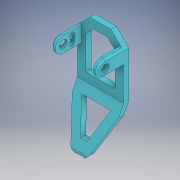
# Autodesk Inventor part: TIBIA
Saved by Autodesk Inventor 2017 (Build 210142000, 142)
## iProperties
Created: 2017-09-24
Part Number: TIBIA
Material: Generic
Document SubType Name: Modeling
Designer: Alexander Miller
Density: 1 g/cm^3
Appearance: Cadet Blue
Author: Alexander Miller
Autodesk Inventor part; units mm, degrees
ref_plane "YZ Plane" through (0, 0, 0) normal (1, 0, 0) x (0, 1, 0)
ref_plane "XZ Plane" through (0, 0, 0) normal (0, 1, 0) x (-1, 0, 0)
ref_plane "XY Plane" through (0, 0, 0) normal (0, 0, 1) x (1, 0, 0)
sketch "Sketch7" plane through (0, 0, 0) normal (0, 1, 0) x (-1, 0, 0)
  line L0 (-15, 22) -> (15, 22)
  line L1 (15, 22) -> (15, -22)
  line L2 (15, -22) -> (-15, -22)
  line L3 (-15, -22) -> (-15, 22)
  line L4 (-10, 18) -> (15, 18)
  line L5 (15, 18) -> (15, -18)
  line L6 (15, -18) -> (-10, -18)
  line L7 (-10, -18) -> (-10, 18)
  point P0 (0, 0)
  point P1 (0, -22)
  point P2 (15, 0)
  point P3 (15, 0)
  dimension "d32" = 4
  dimension "d33" = 5
  dimension "d35" = 44
  dimension "d36" = 25
  constraints: 16 end point, 4 parallel, 3 midpoint, 2 horizontal, 2 horizontal alignment, 2 perpendicular, 1 collinear, 1 vertical alignment
  measures "d32" distance between parallel lines of L0 L4
  measures "d33" distance between parallel lines of L3 L7
  measures "d35" distance of L0.end L1.end
  measures "d36" distance between parallel lines of L7 L1
extrude "Extrusion7" add sketch "Sketch7" along normal blind 15 contours L0 L1 L4 L7 L6 L2 L3
fillet "Fillet4" radius 7.5 4 edges at (-15, 15, 20) (-15, 15, -20) (-15, 0, 20) (-15, 0, -20)
sketch "Sketch8" plane through (15, 0, 22) normal (0, 0, 1) x (1, 0, 0)
  circle A0 centre (-22.5, 7.5) radius 3.675
  arc A1 (-22.5, 15) -> (-22.5, 0) centre (-22.5, 7.5) ccw projected
  point P0 (-15, 0)
  dimension "d40" = 7.35
  constraints: 1 centre point, 1 concentric
  measures "d40" diameter of A0
extrude "Extrusion8" cut sketch "Sketch8" against normal up to surface (4 mm away)
sketch "Sketch9" plane through (15, 0, -22) normal (0, 0, -1) x (-1, 0, 0)
  circle A0 centre (22.5, 7.5) radius 3.75
  arc A1 (22.5, 0) -> (22.5, 15) centre (22.5, 7.5) ccw projected
  point P0 (15, 0)
  dimension "d43" = 7.5
  constraints: 1 centre point, 1 concentric
  measures "d43" diameter of A0
extrude "Extrusion9" cut sketch "Sketch9" against normal up to surface (4 mm away)
sketch "Sketch10" plane through (15, 0, -22) normal (0, 0, -1) x (-1, 0, 0)
  line L0 (22.5, 3.75) -> (5.5, 3.75)
  line L1 (5.5, 3.75) -> (5.5, 11.25)
  line L2 (5.5, 11.25) -> (22.5, 11.25)
  circle A0 centre (22.5, 7.5) radius 3.75 projected
  point P0 (15, 0)
  dimension "d47" = 17
  constraints: 6 end point, 2 perpendicular, 2 point on circle, 2 tangent, 1 horizontal
  measures "d47" distance from line of A0.centre L1
extrude "Extrusion10" cut sketch "Sketch10" against normal blind 2 contours L0 L1 L2 A0
fillet "Fillet5" radius 1.75 2 edges at (9.5, 11.25, -21) (9.5, 3.75, -21)
sketch "Sketch12" plane through (15, 0, 22) normal (0, 0, 1) x (1, 0, 0)
  line L0 (-5, 0) -> (-5, 15) projected
  line L1 (0, 0) -> (0, 15) projected
  line L2 (-5, 25) -> (0, 25)
  line L3 (0, 25) -> (0, -30)
  line L4 (0, -30) -> (-5, -30)
  line L5 (-5, -30) -> (-5, 25)
  line L6 (-22.5, 15) -> (0, 15) projected
  line L7 (0, 0) -> (-22.5, 0) projected
  line L8 (-5, -30) -> (-25, -70.9989)
  line L9 (-25, -70.9989) -> (-20, -70.9989)
  line L10 (-20, -70.9989) -> (0, -30)
  arc A0 (-25, -70.9989) -> (-20, -70.9989) centre (-22.5, -72.2184) ccw
  point P0 (-15, 0)
  point P1 (-22.5, -70.9989)
  dimension "d57" = 10
  dimension "d60" = 100
  dimension "d62" = 30
  constraints: 14 end point, 3 parallel, 2 collinear, 2 horizontal, 2 point on circle, 1 centre point, 1 midpoint, 1 perpendicular, 1 tangent
  measures "d57" distance between parallel lines of L6 L2
  measures "d62" distance between parallel lines of L7 L4
extrude "Extrusion11" add sketch "Sketch12" against normal up to surface (44 mm away) contours L7 L3 L4 L5 | L5 L2 L3 L6 | L4 L10 L9 L8 | L9 A0
chamfer "Chamfer8" distance 12 angle 45 2 edges at (12.5, 25, 22) (12.5, 25, -22)
chamfer "Chamfer9" distance 2 angle 45 4 edges at (-14.3736, 10.5007, 22) (1.25, 0, 22) (-14.3736, 10.5007, -22) (1.25, 0, -22)
sketch "Sketch15" plane through (15, -30, 22) normal (1, 0, 0) x (0, 0, -1)
  line L0 (-4.3749, 0) -> (48.3749, 0)
  line L1 (48.3749, 0) -> (48.3749, -54.3582)
  line L2 (48.3749, -54.3582) -> (-4.3749, -54.3582)
  line L3 (-4.3749, -54.3582) -> (-4.3749, 0)
  line L4 (0, 0) -> (44, 0) projected
  circle A0 centre (22, -35) radius 10
  line L5 (-4.3749, 0) -> (12.8511, -39.0371)
  line L6 (48.3749, 0) -> (31.1489, -39.0371)
  line L7 (12, 55) -> (32, 55) projected
  line L8 (0, -45) -> (44, -45) projected
  point P0 (22, 55)
  point P1 (22, 0)
  point P2 (22, 55)
  dimension "d78" = 20
  constraints: 12 end point, 3 midpoint, 3 tangent, 2 parallel, 2 point on circle, 2 vertical alignment, 1 centre point, 1 collinear, 1 horizontal, 1 perpendicular
  measures "d78" diameter of A0
extrude "Extrusion13" cut sketch "Sketch15" against normal through all contours L5 A0 L6 L1 L2 L3
sketch "Sketch16" plane through (15, -30, 22) normal (1, 0, 0) x (0, 0, -1)
  line L0 (32, 55) -> (44, 43) projected
  line L1 (12, 55) -> (32, 55) projected
  line L2 (0, 43) -> (12, 55) projected
  line L3 (0, 0) -> (0, 43) projected
  line L4 (0, 0) -> (44, 0) projected
  line L5 (44, 0) -> (44, 43) projected
  line L6 (31.1489, -39.0371) -> (44, -9.9143) projected
  line L7 (44, -9.9143) -> (44, 0) projected
  line L8 (0, 0) -> (44, 0) projected
  line L9 (0, -9.9143) -> (0, 0) projected
  line L10 (0, -9.9143) -> (12.8511, -39.0371) projected
  arc A0 (12.8511, -39.0371) -> (13.9991, -40.9989) centre (22, -35) ccw projected
  line L11 (13.9991, -40.9989) -> (30.0009, -40.9989) projected
  arc A1 (30.0009, -40.9989) -> (31.1489, -39.0371) centre (22, -35) ccw projected
  line L12 (15.3137, 47) -> (28.6863, 47)
  line L13 (28.6863, 47) -> (36, 39.6863)
  line L14 (36, 39.6863) -> (36, 8)
  line L15 (36, 8) -> (8, 8)
  line L16 (8, 8) -> (8, 39.6863)
  line L17 (8, 39.6863) -> (15.3137, 47)
  line L18 (18.9309, -32.9989) -> (8, -8.2276)
  line L19 (8, -8.2276) -> (8, -8)
  line L20 (8, -8) -> (36, -8)
  line L21 (36, -8) -> (36, -8.2276)
  line L22 (36, -8.2276) -> (25.0691, -32.9989)
  line L23 (25.0691, -32.9989) -> (18.9309, -32.9989)
  line L24 (8, 8) -> (36, 8)
  line L25 (36, 8) -> (36, -8)
  line L26 (36, -8) -> (8, -8)
  line L27 (8, -8) -> (8, 8)
  point P0 (22, 30)
  dimension "d81" = 8
  constraints: 32 end point, 4 collinear, 2 parallel, 1 horizontal, 1 perpendicular, 1 vertical alignment, 10 other
  measures "d81" distance between parallel lines of L3 L16
extrude "Extrusion14" cut sketch "Sketch16" against normal through all contours L15 L16 L17 L12 L13 L14 | L21 L22 L23 L18 L19 L20
sketch "Sketch17" plane through (10, 0, 18) normal (0, 0, -1) x (-1, 0, 0)
  circle A0 centre (17.5, 7.5) radius 2.675
  circle A1 centre (17.5, 7.5) radius 3.675 projected
  point P0 (10, 0)
  dimension "d84" = 1
  constraints: 1 centre point, 1 concentric
  measures "d84" radial gap between concentric circles of A1 A0
extrude "Extrusion15" add sketch "Sketch17" against normal blind 1
sketch "Sketch18" plane through (10, 0, -18) normal (0, 0, 1) x (1, 0, 0)
  arc A0 (-17.5, 3.75) -> (-17.5, 11.25) centre (-17.5, 7.5) ccw projected
  arc A1 (-8.8762, 4.925) -> (-8.8762, 10.075) centre (-17.5, 7.5) ccw construction
  arc A2 (-7.7504, 4.5888) -> (-7.7504, 10.4112) centre (-17.5, 7.5) ccw
  arc A3 (-10.0021, 5.2612) -> (-10.0021, 9.7388) centre (-17.5, 7.5) ccw
  arc A4 (-10.0021, 5.2612) -> (-7.7504, 4.5888) centre (-8.8762, 4.925) ccw
  arc A5 (-7.7504, 10.4112) -> (-10.0021, 9.7388) centre (-8.8762, 10.075) ccw
  line L0 (-17.5, 3.75) -> (-2.25, 3.75) projected
  line L1 (-2.25, 11.25) -> (-17.5, 11.25) projected
  point P0 (-10, 0)
  point P1 (-8.5, 7.5)
  dimension "d87" = 9
  dimension "d88" = 2.35
  constraints: 11 point on circle, 5 centre point, 5 tangent, 1 coincident, 1 horizontal alignment
  measures "d87" distance of A1.centre point (-8.5, 7.5)
  measures "d88" radial gap between concentric circles of A2 A3
extrude "Extrusion16" cut sketch "Sketch18" against normal through all contours A4 A3 A5 A2
sketch "Sketch19" plane through (10, 0, -18) normal (0, 0, 1) x (1, 0, 0)
  circle A0 centre (-17.5, 7.5) radius 3.75 projected
  arc A1 (-9.2852, 3.8235) -> (-9.2852, 11.1765) centre (-17.5, 7.5) ccw construction
  arc A2 (-7.2999, 2.935) -> (-7.2999, 12.065) centre (-17.5, 7.5) ccw
  arc A3 (-11.2704, 4.712) -> (-11.2704, 10.288) centre (-17.5, 7.5) ccw
  arc A4 (-11.2704, 4.712) -> (-7.2999, 2.935) centre (-9.2852, 3.8235) ccw
  arc A5 (-7.2999, 12.065) -> (-11.2704, 10.288) centre (-9.2852, 11.1765) ccw
  arc A6 (-10.0021, 5.2612) -> (-10.0021, 9.7388) centre (-17.5, 7.5) ccw projected
  arc A7 (-7.7504, 10.4112) -> (-10.0021, 9.7388) centre (-8.8762, 10.075) ccw projected
  arc A8 (-7.7504, 4.5888) -> (-7.7504, 10.4112) centre (-17.5, 7.5) ccw projected
  arc A9 (-10.0021, 5.2612) -> (-7.7504, 4.5888) centre (-8.8762, 4.925) ccw projected
  arc A10 (-10.0021, 5.2612) -> (-10.0021, 9.7388) centre (-17.5, 7.5) ccw projected
  circle A11 centre (-17.5, 7.5) radius 3.75 projected
  arc A12 (-17.5, 15) -> (-17.5, 0) centre (-17.5, 7.5) ccw projected
  line L0 (0, 0) -> (-17.5, 0) projected
  line L1 (0, 0) -> (0, 15) projected
  line L2 (-17.5, 15) -> (0, 15) projected
  arc A13 (-7.7504, 10.4112) -> (-10.0021, 9.7388) centre (-8.8762, 10.075) ccw construction
  arc A14 (-10.0021, 5.2612) -> (-7.7504, 4.5888) centre (-8.8762, 4.925) ccw construction
  point P0 (-10, 0)
  dimension "d91" = 4.35
  constraints: 13 point on circle, 5 centre point, 4 tangent, 1 coincident
  measures "d91" radial gap between concentric circles of A2 A3
extrude "Extrusion17" cut sketch "Sketch19" against normal blind 1 contours A4 A3 A5 A2
body "Solid2"
